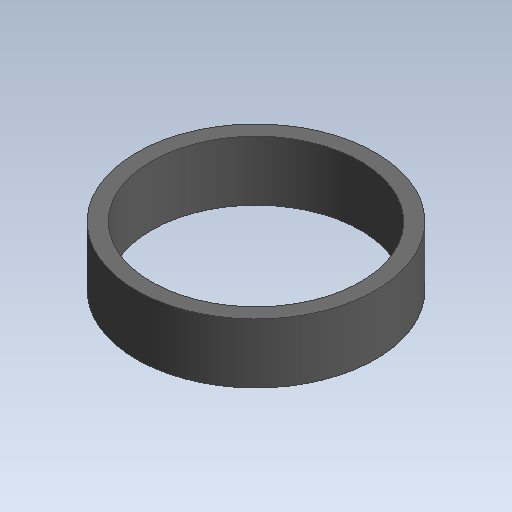
# Autodesk Inventor part: オイレスd14D16L4
Saved by Autodesk Inventor 2020.2 (Build 242310000, 310)
## iProperties
Part Number: オイレスd14D16L4
Material: 一般
Catalog Web Link: www.cadenas.de
Description: Flange Bushings-80F
Vendor: OILES
Document SubType Name: Modeling
Designer: partserver
Manufacturer: OILES
Mass: 0.188496 g
Surface Area: 4.71239 cm^2
Volume: 0.188496 cm^3
Density: 1 g/cm^3
Appearance: PSOLRGB-127-127-127
Category: PARTsolutions
Company: OILES
PSOL_IDENT_0: {$CADENAS_DATA\23d-libs\oiles\plastic_bearings\oiles_80\flange_bushings_80b.prj},166 {VTYP=3D},{NB=8
PSOL_IDENT_1: 0F-0603},{LINA=80F-0603},{NN=Flange Bushings},{DATE=15.04.2019 22:54:28},{GEOMDATE=07.11.2016 06:24:
PSOL_IDENT_2: 13},{VERSION=},{LINEID=170},{WBVAR=},{WBNUMERIC=}  {NB=80F-0603},{LINA=80F-0603},{KT=DUMMY},{ORDERNO=
PSOL_IDENT_3: 80F-0603},{S=6},{SRT=h7(0/-0.012)},{H=8},{HRT=H7(+0.015/0)},{ID=6},{IDT=+0.095/+0.045},{OD=8},{ODT=+
PSOL_IDENT_4: 0.157/+0.045},{F=12},{FT=1.0},{FTT=0/-0.10},{L=3},{LT=0/-0.3},{A=0.3},{B=1.0},{C=C0.3},{CC=0.300},{C
PSOL_IDENT_5: R=0.000},{TE=-40~80°C},{P=17.5N/mm2  (179kgf/cm2)},{V=0.85m/s  (51m/min)},{PV=2.45N/mm2•m/s  (1,500k
PSOL_IDENT_6: gf/cm2•m/min)},{AIT=The inner diameter tolerances are the values after pressing into a ring gauge of
PSOL_IDENT_7: OD+-0.002},{CAU=Please refer to catalog about detail.}
NB: 80F-0603
NN: Flange Bushings
NT: 80F
NBSYN: $ORDERNO.
LINA: 80F-0603
CATALOG: OILES CORPORATION
ORDERNO: 80F-0603
S: 6
SRT: h7(0/-0.012)
H: 8
HRT: H7(+0.015/0)
ID: 6
IDT: +0.095/+0.045
OD: 8
ODT: +0.157/+0.045
F: 12
FT: 1
FTT: 0/-0.10
L: 3
LT: 0/-0.3
TE: -40~80°C
P: 17.5N/mm2  (179kgf/cm2)
V: 0.85m/s  (51m/min)
PV: 2.45N/mm2•m/s  (1,500kgf/cm2•m/min)
AIT: The inner diameter tolerances are the values after pressing into a ring gauge of OD+-0.002.
CAU: Please refer to catalog about detail.
SUPPLIER: OILES
ARTICLENO: 80F-0603
BOMINFO: 80F-0603
CREATOR: CADENAS GmbH
Title: 80F-0603
Author: Cadenas PARTsolutions
Comments: 80F
Autodesk Inventor part; units mm, degrees
ref_plane "YZ Plane" through (0, 0, 0) normal (1, 0, 0) x (0, 1, 0)
ref_plane "XZ Plane" through (0, 0, 0) normal (0, 1, 0) x (-1, 0, 0)
ref_plane "XY Plane" through (0, 0, 0) normal (0, 0, 1) x (1, 0, 0)
sketch "Sketch_1" plane through (0, 0, 0) normal (0, 0, 1) x (1, 0, 0)
  circle A0 centre (0, 0) radius 8
  circle A1 centre (0, 0) radius 7
  dimension "d9" = 16
  dimension "d10" = 14
  constraints: 2 centre point, 1 coincident
  measures "d9" diameter of A0
  measures "d10" diameter of A1
extrude "押し出し1" add sketch "Sketch_1" along normal blind 4
